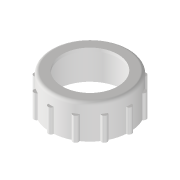
# Autodesk Inventor part: 00_Compression_Coupling_3inch_KingBrothers_CPC-3000_locking
Saved by Autodesk Inventor 2022 (Build 260153000, 153)
## iProperties
Created: 2022-04-19
Part Number: 00_Compression_Coupling_3inch_KingBrothers_CPC-3000_locking
Material: Generic
Document SubType Name: Modeling
Designer: Prakash Lab
Density: 1 g/cm^3
Appearance: Default
Author: Prakash Lab
Autodesk Inventor part; units mm, degrees
ref_plane "YZ Plane" through (0, 0, 0) normal (1, 0, 0) x (0, 1, 0)
ref_plane "XZ Plane" through (0, 0, 0) normal (0, 1, 0) x (-1, 0, 0)
ref_plane "XY Plane" through (0, 0, 0) normal (0, 0, 1) x (1, 0, 0)
sketch "Sketch1" plane through (0, 0, 0) normal (0, 1, 0) x (-1, 0, 0)
  circle A0 centre (0, 0) radius 63.465
  circle A1 centre (0, 0) radius 55.575
  dimension "d0" = 126.93
  dimension "d1" = 111.15
  constraints: 2 centre point, 2 coincident
  measures "d0" diameter of A0
  measures "d1" diameter of A1
extrude "Extrusion1" add sketch "Sketch1" along normal blind 55.37
sketch "Sketch2" plane through (0, 55.37, 0) normal (0, 1, 0) x (1, 0, 0)
  circle A0 centre (0, 0) radius 63.465 projected
  circle A1 centre (0, 0) radius 45.115
  dimension "d4" = 90.23
  constraints: 1 centre point, 1 coincident
  measures "d4" diameter of A1
extrude "Extrusion2" add sketch "Sketch2" against normal blind 5
fillet "Fillet1" radius 5 1 edges at (63.465, 55.37, 0)
sketch "Sketch3" plane through (0, 0, 0) normal (0, -1, 0) x (1, 0, 0)
  circle A0 centre (0, 0) radius 63.465 projected
  circle A1 centre (63.465, 0) radius 4.5231
  constraints: 1 centre point, 1 horizontal alignment, 1 other
extrude "Extrusion3" add sketch "Sketch3" against normal blind 37.92 contours A0 A1 | A0 A1 picked at (62.045, -1.0257) picked at (64.8107, -1.1706)
pattern_circular "Circular Pattern1" count 12 over 360 about axis through (0, 0, 0) along (0, 1, 0) of "Extrusion3"
body "Solid1"
